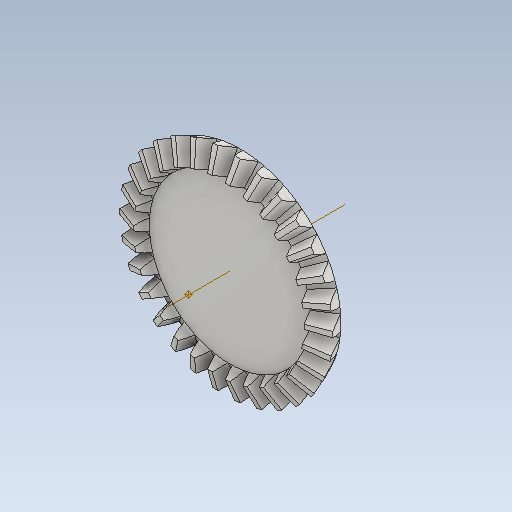
# Autodesk Inventor part: Kegelrad2
Saved by Autodesk Inventor 2021 (Build 250183000, 183)
## iProperties
Created: 2021-01-22
Part Number: Kegelrad2
Material: Steel, Mild
Document SubType Name: Modeling
Designer: LETPJG
Categories: <?xml version="1.0" encoding="UTF-16"?> <MemberInstance><Categories><FamilyTemplate><FamilyTemplateParameter ValueType="xs:double" Id="1" ObjectReferenceKey="da_z" ObjectType="kUserParameterObject"/><FamilyTemplateParameter ValueType="xs:double" Id="2" ObjectReferenceKey="da_b" ObjectType="kUserParameterObject"/><FamilyTemplateParameter ValueType="xs:double" Id="3" ObjectReferenceKey="da_beta" ObjectType="kUserParameterObject"/><FamilyTemplateParameter ValueType="xs:double" Id="4" ObjectReferenceKey="da_dae" ObjectType="kUserParameterObject"/><FamilyTemplateParameter ValueType="xs:double" Id="5" ObjectReferenceKey="da_ve" ObjectType="kUserParameterObject"/><FamilyTemplateParameter ValueType="xs:double" Id="6" ObjectReferenceKey="da_omega" ObjectType="kUserParameterObject"/><FamilyTemplateParameter ValueType="xs:string" Id="7" ObjectReferenceKey="EAIAABAAAAAAHwAAAAAAAIAAAAAAAAAA" ObjectType="83914240" SubObjectId="SurfaceGeometry"/></FamilyTemplate><ParamToTemplateMap><ParamToTemplate CategoryParameter="//CategoryParameter[@InternalName='046C89C9-8512-4d59-83FE-43B91F4F132A']" TemplateParameter="1"/><ParamToTemplate CategoryParameter="//CategoryParameter[@InternalName='2552DF32-E462-4b46-AEBF-C6C7768E72AC']" TemplateParameter="2"/><ParamToTemplate CategoryParameter="//CategoryParameter[@InternalName='C9EE641D-15FC-4fae-A226-E94C4372FDD7']" TemplateParameter="3"/><ParamToTemplate><ParamToTemplate CategoryParameter="//CategoryParameter[@InternalName='00B6519A-459B-49c7-AD84-2E56D39A5744']" ConstantValue="-0.000000"/></ParamToTemplate><ParamToTemplate><ParamToTemplate CategoryParameter="//CategoryParameter[@InternalName='04B31F0E-C7A6-4894-AA32-9629BEFACF47']" ConstantValue="1.000000"/></ParamToTemplate><ParamToTemplate><ParamToTemplate CategoryParameter="//CategoryParameter[@InternalName='43CBEC2E-7847-49e7-A936-2F7889FCB2D9']" ConstantValue="0.200000"/></ParamToTemplate><ParamToTemplate><ParamToTemplate CategoryParameter="//CategoryParameter[@InternalName='B1EFC894-105D-4ebd-86BF-FA20ED196853']" ConstantValue="0.300000"/></ParamToTemplate><ParamToTemplate><ParamToTemplate CategoryParameter="//CategoryParameter[@InternalName='51175063-3D10-4879-93E8-6246FE8B403D']" ConstantValue="2060000000.000000"/></ParamToTemplate><ParamToTemplate><ParamToTemplate CategoryParameter="//CategoryParameter[@InternalName='A3A52E27-4454-46a9-B0BD-C932399B70AF']" ConstantValue="0.300000"/></ParamToTemplate><ParamToTemplate CategoryParameter="//CategoryParameter[@InternalName='2A200944-5A8C-41ca-B96E-8520D2E510F1']" TemplateParameter="4"/><ParamToTemplate><ParamToTemplate CategoryParameter="//CategoryParameter[@InternalName='1A637F62-92C8-44bc-B81F-10802510B579']" ConstantValue="4.934602"/></ParamToTemplate><ParamToTemplate CategoryParameter="//CategoryParameter[@InternalName='B52DD4BE-6863-48fb-BF58-89EF6F9EC65C']" TemplateParameter="5"/><ParamToTemplate><ParamToTemplate CategoryParameter="//CategoryParameter[@InternalName='3956BFF2-84D2-457d-93C2-9B0613DEBA67']" ConstantValue="0.894527"/></ParamToTemplate><ParamToTemplate CategoryParameter="//CategoryParameter[@InternalName='739CFA02-461B-4bf8-8049-181FCAD8B28F']" TemplateParameter="6"/><ParamToTemplate><ParamToTemplate CategoryParameter="//CategoryParameter[@InternalName='A27E999F-E2CE-4481-8A2A-EBF499C4C3C5']" ConstantValue="-0.000000"/></ParamToTemplate><ParamToTemplate><ParamToTemplate CategoryParameter="//CategoryParameter[@InternalName='9E1B4470-B2D3-4ff1-B813-535BB4CDF51A']" ConstantValue="3520000.000000"/></ParamToTemplate><ParamToTemplate><ParamToTemplate CategoryParameter="//CategoryParameter[@InternalName='F8452263-BFF6-458c-9FB1-07C4B99E95CD']" ConstantValue="11400000.000000"/></ParamToTemplate><ParamToTemplate><ParamToTemplate CategoryParameter="//CategoryParameter[@InternalName='3E3BB259-FD49-497f-8171-6EBC954A3479']" ConstantValue="2.000000"/></ParamToTemplate><ParamToTemplate CategoryParameter="//CategoryParameter[@InternalName='27C3BAF2-7550-4e4b-AE2C-0DB134B7D9B7']" TemplateParameter="7"/></ParamToTemplateMap><Category DisplayName="Gear" InternalName="DC85795E-93AB-48d5-8EEE-5A27447B64BD" Mnemonic="Gear"><CategoryParameter DisplayName="z" InternalName="046C89C9-8512-4d59-83FE-43B91F4F132A" Mnemonic="z"/><CategoryParameter DisplayName="b" InternalName="2552DF32-E462-4b46-AEBF-C6C7768E72AC" Mnemonic="b"/><CategoryParameter DisplayName="||b|" InternalName="C9EE641D-15FC-4fae-A226-E94C4372FDD7" Mnemonic="beta"/><CategoryParameter DisplayName="x" InternalName="00B6519A-459B-49c7-AD84-2E56D39A5744" Mnemonic="x"/><CategoryParameter DisplayName="a*" InternalName="04B31F0E-C7A6-4894-AA32-9629BEFACF47" Mnemonic="a"/><CategoryParameter DisplayName="c*" InternalName="43CBEC2E-7847-49e7-A936-2F7889FCB2D9" Mnemonic="c"/><CategoryParameter DisplayName="r|.f|*" InternalName="B1EFC894-105D-4ebd-86BF-FA20ED196853" Mnemonic="rf"/><CategoryParameter DisplayName="E" InternalName="51175063-3D10-4879-93E8-6246FE8B403D" Mnemonic="E"/><CategoryParameter DisplayName="||m|" InternalName="A3A52E27-4454-46a9-B0BD-C932399B70AF" Mnemonic="mi"/><Category DisplayName="BevelGear" InternalName="0C98F69A-0C2B-4791-B2FE-7691BB227E77" Mnemonic="BevelGear"><CategoryParameter DisplayName="d|.ae|" InternalName="2A200944-5A8C-41ca-B96E-8520D2E510F1" Mnemonic="dae"/><CategoryParameter DisplayName="d|.ai|" InternalName="1A637F62-92C8-44bc-B81F-10802510B579" Mnemonic="dai"/><CategoryParameter DisplayName="A|.e|" InternalName="B52DD4BE-6863-48fb-BF58-89EF6F9EC65C" Mnemonic="ve"/><CategoryParameter DisplayName="A|.i|" InternalName="3956BFF2-84D2-457d-93C2-9B0613DEBA67" Mnemonic="vi"/><CategoryParameter DisplayName="||S|" InternalName="739CFA02-461B-4bf8-8049-181FCAD8B28F" Mnemonic="omega"/><CategoryParameter DisplayName="x|.t|" InternalName="A27E999F-E2CE-4481-8A2A-EBF499C4C3C5" Mnemonic="xt"/><CategoryParameter DisplayName="||s||.Flim|" InternalName="9E1B4470-B2D3-4ff1-B813-535BB4CDF51A" Mnemonic="sFlim"/><CategoryParameter DisplayName="||s||.Hlim|" InternalName="F8452263-BFF6-458c-9FB1-07C4B99E95CD" Mnemonic="sHlim"/><CategoryParameter DisplayName="Typ" InternalName="3E3BB259-FD49-497f-8171-6EBC954A3479" Mnemonic="type"/><CategoryParameter DisplayName="PitchDiameter" InternalName="27C3BAF2-7550-4e4b-AE2C-0DB134B7D9B7" Mnemonic="IDS_PITCHDIAM"/></Category></Category></Categories></MemberInstance>
Mass: 60.9118 g
Surface Area: 34.3074 cm^2
Volume: 7.7496 cm^3
Density: 7.86 g/cm^3
Appearance: Steel
CustomPartVersion: 1
Author: LETPJG
Autodesk Inventor part; units mm, degrees
ref_plane "Netzebene2" through (0, 0, 0) normal (0.9945219, 0.1045285, 0) x (0, 0, 1)
sketch "Skizze des Zahnradkörpers" plane through (0, 0, 0) normal (1, 0, 0) x (0, 1, 0)
  line L0 (0, 0) -> (29.045742, -15.202133) construction
  line L1 (29.045742, -15.202133) -> (30.795215, -11.164889)
  line L2 (30.795215, -11.164889) -> (0, 0) construction
  line L3 (30, -13) -> (0, 0) construction
  line L4 (23.271341, -12.179893) -> (24.673012, -8.945267)
  line L5 (29.045742, -15.202133) -> (23.271341, -12.179893)
  line L6 (30.795215, -11.164889) -> (24.673012, -8.945267)
  line L7 (0, -39.386751) -> (0, 6.564458)
  line L8 (0, -13) -> (30.795215, -13) construction
  dimension "d0" = 60
  dimension "d1" = 58.09148
  dimension "d2" = 61.59043
  dimension "d3" = 6.5
  dimension "d4" = 11.16489
  constraints: 16 end point, 4 point on line, 3 perpendicular, 2 collinear, 1 horizontal alignment, 1 vertical alignment
  measures "d0" diameter of L3.start L7
  measures "d1" diameter of L0.end L7
  measures "d2" diameter of L1.end L7
  measures "d3" distance between parallel lines of L1 L4
  measures "d4" vertical distance of L1.end L0.start
revolve "Zahnradkörper" add sketch "Skizze des Zahnradkörpers" angle 360 about axis through (0, 0, 0) along (0, 0, 1)
ref_plane "Zahnebene" through (0, 30, -13) normal (0, -0.9175556, 0.3976074) x (1, 0, 0)
sketch "Startskizze" plane through (0, 30, -13) normal (0, -0.9175556, 0.3976074) x (1, 0, 0)
  line L0 (0, -23.505131) -> (0, 10.644758)
  arc A0 (-0.675829, -2.928) -> (-3.087918, 3.259452) centre (-26.376916, -9.383313) ccw
  arc A1 (3.087918, 3.259452) -> (0.675829, -2.928) centre (26.376916, -9.383313) ccw
  line L1 (-0.675829, -2.928) -> (0.675829, -2.928)
  arc A2 (3.087918, 3.259452) -> (-3.087918, 3.259452) centre (0, -75.451305) ccw
  dimension "d7" = 26.49938
  dimension "d8" = 26.37692
  dimension "d9" = 66.06799
  dimension "d57" = 78.7713
  dimension "d58" = 72.5233
  constraints: 6 point on circle, 3 centre point, 3 symmetric about line, 2 end point, 1 coincident, 1 perpendicular, 1 other
  measures "d7" radius of A0
  measures "d8" horizontal distance of point (0, -75.451) A0.centre
  measures "d9" vertical distance of point (0, -75.451) A0.centre
  measures "d57" radius of A2
  measures "d58" distance from line of A2.centre L1
ref_plane "Endebene" through (0, 23.834026, -10.328078) normal (0, -0.9175556, 0.3976074) x (1, 0, 0)
sketch "Endskizze" plane through (0, 23.834026, -10.328078) normal (0, -0.9175556, 0.3976074) x (1, 0, 0)
  line L0 (0, -15.35404) -> (0, 6.953444)
  arc A0 (-0.536924, -2.326201) -> (-2.453251, 2.589529) centre (-20.955604, -7.454738) ccw
  arc A1 (2.453251, 2.589529) -> (0.536924, -2.326201) centre (20.955604, -7.454738) ccw
  line L1 (-0.536924, -2.326201) -> (0.536924, -2.326201)
  arc A2 (2.453251, 2.589529) -> (-2.453251, 2.589529) centre (0, -59.943613) ccw
  dimension "d12" = 21.05289
  dimension "d15" = 20.9556
  dimension "d16" = 52.48887
  dimension "d59" = 62.58124
  dimension "d60" = 57.61741
  constraints: 6 point on circle, 3 centre point, 3 symmetric about line, 2 end point, 1 coincident, 1 other
  measures "d12" radius of A0
  measures "d15" horizontal distance of A0.centre point (0, -59.944)
  measures "d16" vertical distance of A0.centre point (0, -59.944)
  measures "d59" radius of A2
  measures "d60" distance from line of A2.centre L1
loft "Loft" cut profiles "Startskizze", "Endskizze"
pattern_circular "Circular Pattern" count 30 over 360 about axis through (0, 0, 0) along (0, 0, 1) of "Loft"
sketch3d "3D-Skizze rechts"
ref_plane "Endebene rechts" through (-2.1547, 23.736429, -10.328078) normal (0.082951, -0.9137984, 0.3976074) x (0.9959051, 0.0904044, 0)
sketch "Endskizze rechts" plane through (-2.1547, 23.736429, -10.328078) normal (0.082951, -0.9137984, 0.3976074) x (0.9959051, 0.0904044, 0)
  arc A0 (-0.536924, -2.326201) -> (-2.453251, 2.589529) centre (-20.955604, -7.454738) ccw
  line L0 (0, -73.346068) -> (0, 17.16911)
  arc A1 (2.453251, 2.589529) -> (0.536924, -2.326201) centre (20.955604, -7.454738) ccw
  line L1 (-0.536924, -2.326201) -> (0.536924, -2.326201)
  arc A2 (2.453251, 2.589529) -> (-2.453251, 2.589529) centre (0, -59.943613) ccw
  dimension "d70" = 20.9556
  dimension "d71" = 52.48887
  dimension "d72" = 21.05289
  dimension "d73" = 57.61741
  dimension "d74" = 62.58124
  constraints: 6 point on circle, 3 centre point, 3 symmetric about line, 2 end point, 1 coincident, 1 perpendicular, 1 other
  measures "d70" horizontal distance of A2.centre A0.centre
  measures "d71" vertical distance of point (0, -59.944) A0.centre
  measures "d72" radius of A0
  measures "d73" distance from line of point (0, -59.944) L1
  measures "d74" radius of A2
feature "Erhebung rechts" [suppressed]
pattern_circular "Runde Anordnung rechts" [suppressed]
sketch3d "3D-Skizze links"
ref_plane "Endebene links" through (2.196628, 23.736429, -10.362439) normal (-0.0845092, -0.913194, 0.3986664) x (0.9957453, -0.0921487, 0)
sketch "Endskizze links" plane through (2.196628, 23.736429, -10.362439) normal (-0.0845092, -0.913194, 0.3986664) x (0.9957453, -0.0921487, 0)
  line L0 (0, -73.996889) -> (0, 17.852264)
  arc A0 (-0.536924, -2.296174) -> (-2.453251, 2.619556) centre (-20.955604, -7.424711) ccw
  arc A1 (2.453251, 2.619556) -> (0.536924, -2.296174) centre (20.955604, -7.424711) ccw
  line L1 (-0.536924, -2.296174) -> (0.536924, -2.296174)
  ellipse E0 centre (0, -8.203669) end of major axis (24.673012, -8.203669) minor radius 9.836301
  arc A2 (2.453251, 2.619556) -> (-2.453251, 2.619556) centre (0, -59.913586) ccw
  dimension "d56" = 9.8363
  dimension "d30" = 21.05289
  dimension "d31" = 20.9556
  dimension "d32" = 52.48887
  dimension "d61" = 62.58124
  dimension "d62" = 57.61741
  constraints: 6 point on circle, 3 centre point, 3 symmetric about line, 2 end point, 1 coincident, 2 other
  measures "d30" radius of A0
  measures "d31" horizontal distance of point (0, -59.914) A0.centre
  measures "d32" vertical distance of A0.centre point (0, -59.914)
  measures "d61" radius of A2
  measures "d62" distance from line of point (0, -59.914) L1
feature "Erhebung links" [suppressed]
pattern_circular "Runde Anordnung links" [suppressed]
sketch "Körperskizze" plane through (0, 0, 0) normal (1, 0, 0) x (0, 1, 0)
  line L0 (0, -35.037536) -> (0, -19.530831)
  line L1 (29.045742, -15.202133) -> (23.271341, -12.179893)
  line L2 (23.271341, -12.179893) -> (0, -12.179893)
  line L3 (29.045742, -15.202133) -> (0, -15.202133)
  constraints: 4 end point, 2 perpendicular, 2 point on line
sketch "Körperskizze outline for Festkörper" plane through (0, 0, 0) normal (1, 0, 0) x (0, 1, 0)
  line L0 (0, -15.202133) -> (29.045742, -15.202133)
  line L1 (0, -12.179893) -> (0, -15.202133)
  line L2 (23.271341, -12.179893) -> (0, -12.179893)
  line L3 (29.045742, -15.202133) -> (23.271341, -12.179893)
revolve "Festkörper" add sketch "Körperskizze outline for Festkörper" angle 360 about axis through (0, 0, 0) along (0, 0, 1)
sketch "Sketch6" plane through (0, 0, 0) normal (1, 0, 0) x (0, 1, 0)
  line L0 (30, -13) -> (0, 0)
  line L1 (0, -37.799919) -> (0, 6.299986)
surface revolve "Flankendurchmesser" sketch "Sketch6" angle 360 about axis through (0, 0, 0) along (0, 0, 1) shown no curves L0
equation "\"d0\" = da_de"
equation "\"d1\" = da_dfe"
equation "\"d2\" = da_dae"
equation "\"d3\" = da_b"
equation "\"d4\" = da_ve"
equation "\"d7\" = fd_rr"
equation "\"d8\" = fd_x"
equation "\"d9\" = fd_y"
equation "\"d57\" = 0.5 * fd_dva + 0.3 * da_he"
equation "\"d58\" = 0.5 * fd_dva - 1.12 * da_he"
equation "\"da_teethtype\" = 0"
equation "\"da_b\" = 6.5"
equation "\"da_de\" = 60"
equation "\"da_dae\" = 61.59043"
equation "\"da_dfe\" = 58.09148"
equation "\"da_le\" = 32.69557"
equation "\"da_omega\" = 90deg"
equation "\"da_beta\" = 0"
equation "\"da_delta\" = 66.571307deg"
equation "\"da_alpha\" = 20deg"
equation "\"da_he\" = 4.4"
equation "\"da_ve\" = 11.16489"
equation "\"da_zv\" = 75.451305"
equation "\"fd_loft\" = da_b + 0.05 * da_he"
equation "\"fd_x\" = fd_x1 + fd_x2"
equation "\"fd_y\" = fd_y1 - fd_y2"
equation "\"fd_dd\" = fd_dva - 0.8 * da_he"
equation "\"da_dvw\" = 150.90261"
equation "\"d11\" = fd_loft"
equation "\"da_dm\" = 54.03589"
equation "\"da_x\" = 0"
equation "\"da_m\" = 2"
equation "\"d50\" = da_omega"
equation "\"fd_rr\" = 26.499376"
equation "\"fd_dva\" = 154.90261"
equation "\"fd_x1\" = 1.588132"
equation "\"fd_x2\" = 24.788784"
equation "\"fd_y1\" = 75.434589"
equation "\"fd_y2\" = 9.366598"
body "Solid1"
body "Srf1"
